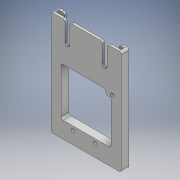
# Autodesk Inventor part: IR Lock Mount
Saved by Autodesk Inventor 2018 (Build 220112000, 112)
## iProperties
Created: 2017-07-06
Part Number: IR Lock Mount
Material: Generic
Document SubType Name: Modeling
Designer: klyu
Density: 1 g/cm^3
Appearance: Default
Author: klyu
Autodesk Inventor part; units mm, degrees
ref_plane "YZ Plane" through (0, 0, 0) normal (1, 0, 0) x (0, 1, 0)
ref_plane "XZ Plane" through (0, 0, 0) normal (0, 1, 0) x (-1, 0, 0)
ref_plane "XY Plane" through (0, 0, 0) normal (0, 0, 1) x (1, 0, 0)
sketch "Sketch1" plane through (0, 0, 0) normal (0, 1, 0) x (-1, 0, 0)
  line L0 (0, 0) -> (4.5, 0)
  line L1 (4.5, 0) -> (4.5, -20)
  line L2 (4.5, -20) -> (0, -20)
  line L3 (0, -20) -> (0, 0)
  line L4 (34, 0) -> (38.5, 0)
  line L5 (38.5, 0) -> (38.5, -20)
  line L6 (38.5, -20) -> (34, -20)
  line L7 (34, -20) -> (34, 0)
  line L8 (51.25, 0) -> (-12.75, 0)
  line L9 (-12.75, 0) -> (-12.75, -25)
  line L10 (-12.75, -25) -> (51.25, -25)
  line L11 (51.25, -25) -> (51.25, 0)
  line L12 (19.25, 0) -> (19.25, -42)
  dimension "d0" = 4.5
  dimension "d1" = 20
  dimension "d2" = 4.5
  dimension "d3" = 20
  dimension "d4" = 38.5
  dimension "d5" = 25
  dimension "d6" = 64
  dimension "d7" = 14.75
  dimension "d8" = 32
  constraints: 26 end point, 6 parallel, 3 horizontal, 3 perpendicular, 2 collinear, 1 midpoint, 1 vertical
  measures "d0" distance between parallel lines of L1 L3
  measures "d1" distance between parallel lines of L2 L0
  measures "d2" distance between parallel lines of L5 L7
  measures "d3" distance between parallel lines of L6 L4
  measures "d4" distance between parallel lines of L3 L5
  measures "d5" distance between parallel lines of L10 L8
  measures "d6" distance between parallel lines of L9 L11
  measures "d7" distance between parallel lines of L12 L7
  measures "d8" distance between parallel lines of L12 L11
extrude "Extrusion1" add sketch "Sketch1" along normal blind 2 contours L3 L2 L1 L8 L12 L10 L9 | L8 L7 L6 L5 L11 L10 L12
sketch "Sketch2" plane through (0, 2, 0) normal (0, 1, 0) x (1, 0, 0)
  line L0 (0, 0) -> (12.75, 0) projected
  line L1 (12.75, 0) -> (10.75, 0)
  line L2 (10.75, 0) -> (10.75, 25)
  line L3 (10.75, 25) -> (12.75, 25)
  line L4 (12.75, 25) -> (12.75, 0)
  line L5 (12.75, 25) -> (-51.25, 25) projected
  line L6 (-49.25, 0) -> (-51.25, 0)
  line L7 (-51.25, 0) -> (-51.25, 25)
  line L8 (-51.25, 25) -> (-49.25, 25)
  line L9 (-49.25, 25) -> (-49.25, 0)
  line L10 (-51.25, 25) -> (-51.25, 0) projected
  line L11 (-51.25, 0) -> (-38.5, 0) projected
  point P0 (13.75, 26)
  dimension "d11" = 2
  dimension "d12" = 2
  constraints: 14 end point, 4 collinear, 3 parallel, 2 horizontal, 2 perpendicular, 1 vertical, 3 other
  measures "d11" distance between parallel lines of L4 L2
extrude "Extrusion2" add sketch "Sketch2" along normal blind 3
sketch "Sketch3" plane through (0, 5, 0) normal (0, 1, 0) x (1, 0, 0)
  line L0 (-51.25, 0) -> (-44.25, 0)
  line L1 (-44.25, 0) -> (-44.25, 25)
  line L2 (-44.25, 25) -> (-51.25, 25)
  line L3 (-51.25, 25) -> (-51.25, 0)
  line L4 (12.75, 0) -> (12.75, 25) projected
  line L5 (12.75, 0) -> (5.75, 0)
  line L6 (5.75, 0) -> (5.75, 25)
  line L7 (5.75, 25) -> (12.75, 25)
  line L8 (12.75, 25) -> (12.75, 0)
  line L9 (10.75, 25) -> (-49.25, 25) projected
  point P0 (0, 0)
  dimension "d15" = 7
  dimension "d16" = 7
  constraints: 16 end point, 4 parallel, 2 horizontal, 2 perpendicular, 1 collinear, 1 point on line
  measures "d15" distance between parallel lines of L3 L1
  measures "d16" distance between parallel lines of L4 L6
extrude "Extrusion3" add sketch "Sketch3" along normal blind 2
sketch "Sketch4" plane through (12.75, 0, -25) normal (0, 0, -1) x (-1, 0, 0)
  line L0 (0, 0) -> (0, 7) projected
  line L1 (0, 7) -> (64, 7)
  line L2 (64, 7) -> (64, 0)
  line L3 (64, 0) -> (0, 0)
  line L4 (0, 0) -> (0, 7)
  line L5 (64, 0) -> (64, 7) projected
  line L6 (0, 0) -> (64, 0) projected
  point P0 (12.75, 0)
  constraints: 8 end point, 2 collinear, 2 parallel, 1 horizontal, 1 perpendicular
extrude "Extrusion4" add sketch "Sketch4" along normal blind 70
sketch "Sketch5" plane through (0, 7, 0) normal (0, 1, 0) x (1, 0, 0)
  line L0 (3.65, 36) -> (-42.15, 36)
  line L1 (-42.15, 36) -> (-42.15, 80)
  line L2 (-42.15, 80) -> (3.65, 80)
  line L3 (3.65, 80) -> (3.65, 36)
  circle A0 centre (-31.15, 83.7) radius 1.65
  line L4 (12.75, 0) -> (12.75, 95) projected
  line L5 (-44.25, 25) -> (5.75, 25) projected
  line L6 (-19.25, 25) -> (-19.25, 95)
  line L7 (12.75, 95) -> (-51.25, 95) projected
  circle A1 centre (4.65, 37.8) radius 1.65
  line L8 (-51.25, 0) -> (-51.25, 95) projected
  circle A2 centre (-11.15, 83.7) radius 1.65
  line L9 (-11.15, 83.7) -> (-31.15, 83.7)
  circle A3 centre (55, 5) radius 1.65
  line L10 (3.65, 40.5) -> (-1.35, 40.5)
  line L11 (-1.35, 40.5) -> (-1.35, 36)
  point P0 (0, 0)
  dimension "d21" = 45.8
  dimension "d22" = 44
  dimension "d23" = 3.3
  dimension "d25" = 15
  dimension "d26" = 3.3
  dimension "d28" = 3.3
  dimension "d30" = 11
  dimension "d31" = 31
  dimension "d32" = 3.7
  dimension "d33" = 3.3
  dimension "d34" = 4.5
  dimension "d35" = 5
  dimension "d36" = 1
  dimension "d37" = 1.8
  constraints: 16 end point, 4 centre point, 3 horizontal, 2 midpoint, 2 parallel, 2 perpendicular, 2 point on line, 1 other
  measures "d21" distance between parallel lines of L1 L3
  measures "d22" distance between parallel lines of L2 L0
  measures "d23" diameter of A0
  measures "d25" distance between parallel lines of L7 L2
  measures "d26" diameter of A1
  measures "d28" diameter of A2
  measures "d30" distance from line of L1 L9.end
  measures "d31" distance from line of L1 L9.start
  measures "d32" distance from line of L9.end L2
  measures "d33" diameter of A3
  measures "d34" distance between parallel lines of L10 L0
  measures "d35" distance between parallel lines of L11 L3
  measures "d36" distance from line of A1.centre L3
  measures "d37" distance from line of L0 A1.centre
extrude "Extrusion5" cut sketch "Sketch5" against normal through all contours L0 L6 L2 L3 L10 L11 | A1 L3 | L3 A1 | L0 L1 L2 L6 | A0 | A2
fillet "Fillet1" radius 2 21 edges at (12.75, 3.5, 0) (0, 1, 0) (-4.5, 1, 0) (-34, 1, 0) (-38.5, 1, 0) (-51.25, 3.5, 0) (-44.25, 6, 0) (5.75, 6, 0) (5.75, 6, -25) (0, 1, -20) (-34, 1, -20) (3.65, 3.5, -80) (-1.35, 3.5, -40.5) (-51.25, 3.5, -95) (-38.5, 1, -20) (-4.5, 1, -20) (-42.15, 3.5, -80) (12.75, 3.5, -95) (-42.15, 3.5, -36) (-1.35, 3.5, -36) (3.65, 3.5, -40.5)
fillet "Fillet2" radius 2 1 edges at (-44.25, 6, -25)
body "Solid1"
